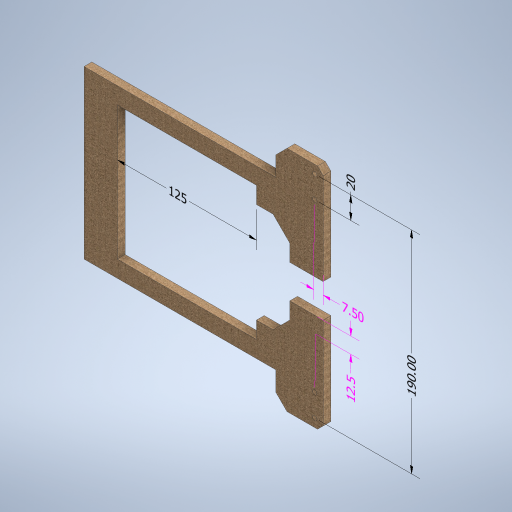
# Autodesk Inventor part: Marco
Saved by Autodesk Inventor 2023.1 (Build 271208000, 208)
## iProperties
Created: 2022-10-28
Part Number: Marco
Material: MDF Medium Density Fiberboard
Document SubType Name: Modeling
Designer: Daniel Peña
Density: 0.8 g/cm^3
Appearance: Cardboard - Corrugated
Author: Daniel Peña
Autodesk Inventor part; units mm, degrees
ref_plane "YZ Plane" through (0, 0, 0) normal (1, 0, 0) x (0, 1, 0)
ref_plane "XZ Plane" through (0, 0, 0) normal (0, 1, 0) x (-1, 0, 0)
ref_plane "XY Plane" through (0, 0, 0) normal (0, 0, 1) x (1, 0, 0)
sketch "Sketch1" plane through (0, 0, 0) normal (0, 0, 1) x (1, 0, 0)
  line L0 (-100, -75) -> (100, -75) projected
  line L1 (100, -75) -> (100, 75) projected
  line L2 (100, 75) -> (-100, 75) projected
  line L3 (-100, 75) -> (-100, -75) projected
  line L4 (-70, -60) -> (55, -60)
  line L5 (55, 60) -> (-70, 60)
  line L6 (-70, 60) -> (-70, 15)
  line L7 (-70, -15) -> (-70, -60)
  line L8 (151.2343, 15) -> (1.2343, 15) projected
  line L9 (1.2343, -15) -> (151.2343, -15) projected
  line L10 (85, -30) -> (85, -15)
  line L11 (85, 15) -> (85, 30)
  line L12 (-100, 75) -> (72.5, 75)
  line L13 (72.5, -75) -> (-100, -75)
  line L14 (-100, -75) -> (-100, 75)
  line L15 (100, -15) -> (85, -15)
  line L16 (100, 15) -> (85, 15)
  line L17 (-100, 0) -> (100, 0) construction
  line L18 (70, 45) -> (70, -45) projected
  line L19 (70, -45) -> (-70, -45) projected
  line L20 (-70, -45) -> (-70, 45) projected
  line L21 (-70, 45) -> (70, 45) projected
  line L22 (-70, 15) -> (-70, -15)
  line L23 (85, -30) -> (70, -45)
  line L24 (70, -45) -> (55, -45)
  line L25 (55, -45) -> (55, -60)
  line L26 (85, 30) -> (70, 45)
  line L27 (70, 45) -> (55, 45)
  line L28 (55, 45) -> (55, 60)
  line L29 (100, -102.5) -> (110, -102.5)
  line L30 (115, -97.5) -> (115, -67.5)
  line L31 (110, -102.5) -> (115, -97.5)
  line L32 (100, -15) -> (115, -15)
  line L33 (115, -67.5) -> (115, -15)
  line L34 (72.5, -75) -> (72.5, -92.5)
  line L35 (82.5, -102.5) -> (100, -102.5)
  line L36 (72.5, -92.5) -> (82.5, -102.5)
  line L37 (100, 102.5) -> (110, 102.5)
  line L38 (115, 97.5) -> (115, 67.5)
  line L39 (110, 102.5) -> (115, 97.5)
  line L40 (100, 15) -> (115, 15)
  line L41 (115, 67.5) -> (115, 15)
  line L42 (72.5, 75) -> (72.5, 92.5)
  line L43 (82.5, 102.5) -> (100, 102.5)
  line L44 (72.5, 92.5) -> (82.5, 102.5)
  point P0 (0, 0)
  point P1 (85, -60)
  point P2 (85, 60)
  point P3 (100, 15)
  point P4 (100, -15)
  point P5 (-70, 15)
  point P6 (85, -22.5)
  point P7 (70, 15)
  point P8 (70, -15)
  point P9 (115, -102.5)
  point P10 (100, -55)
  point P11 (107.5, 75)
  point P12 (107.5, 95)
  point P13 (107.5, -75)
  point P14 (107.5, -95)
  point P15 (72.5, -102.5)
  dimension "d3" = 15
  dimension "d4" = 15
  dimension "d5" = 30
  dimension "d13" = 30
  dimension "d17" = 5
  dimension "d18" = 5
  dimension "d74" = 20
  dimension "d76" = 150
  dimension "d78" = 27.5
  dimension "d79" = 10
  dimension "d80" = 10
  constraints: 70 end point, 15 point on line, 14 symmetric about line, 3 collinear, 3 midpoint, 2 horizontal, 2 perpendicular, 1 parallel, 1 vertical alignment, 3 other
  measures "d3" distance between parallel lines of L1 L11
  measures "d4" distance between parallel lines of L12 L5
  measures "d5" distance between parallel lines of L3 L6
  measures "d13" distance of L5.start point (85, 60)
  measures "d17" distance of L29.end point (115, -102.5)
  measures "d18" distance of L30.start point (115, -102.5)
  measures "d74" distance of point (107.5, 95) point (107.5, 75)
  measures "d76" distance of point (107.5, -75) point (107.5, 75)
  measures "d78" distance of L35.end point (72.5, -102.5)
  measures "d79" distance of L34.end point (72.5, -102.5)
  measures "d80" distance of L35.start point (72.5, -102.5)
extrude "Extrusion1" add sketch "Sketch1" along normal blind 7 contours L3 L2 L1 L8 L11 L26 L21 L28 L5 L6 L20 L7 L4 L25 L19 L23 L10 L9 L0 | L0 L1 L9 L33 L30 L31 L29 L35 L36 L34 | L42 L44 L43 L37 L39 L38 L41 L8 L1 L2
sketch "Sketch2" plane through (0, 0, 7) normal (0, 0, 1) x (1, 0, 0)
  line L0 (-70, -60) -> (-70, 60) construction
  line L1 (-70, 0) -> (130.7679, 0) construction
  line L2 (115, -97.5) -> (115, -15) construction
  line L3 (-100, -102.5) -> (110, -102.5) construction
  line L4 (115, -15) -> (85, -15) construction
  point P0 (0, 0)
  point P1 (107.5, -75)
  point P2 (107.5, -95)
  point P3 (107.5, 75)
  point P4 (107.5, 95)
  point P5 (115, -20)
  point P6 (-100, -75)
  point P7 (110, -15)
  point P8 (115, -20)
  point P9 (100, -15)
  dimension "d21" = 7.5
  dimension "d24" = 7.5
  dimension "d32" = 20
  dimension "d73" = 150
  constraints: 2 end point, 2 symmetric about line, 1 horizontal, 1 midpoint
  measures "d21" distance from line of L2 point (107.5, -95)
  measures "d24" distance from line of L2 point (107.5, -75)
  measures "d32" distance of point (107.5, -95) point (107.5, -75)
  measures "d73" distance of point (107.5, -75) point (107.5, 75)
hole "Hole1" at (107.5, -75, 7) at (107.5, -95, 7) at (107.5, 75, 7) at (107.5, 95, 7) direction (0, 0, -1) diameter 4 end through all
body "Solid1"
